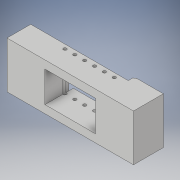
# Autodesk Inventor part: AndersonA
Saved by Autodesk Inventor 2018 (Build 220112000, 112)
## iProperties
Created: 2017-09-11
Part Number: AndersonA
Material: Generic
Document SubType Name: Modeling
Designer: Srinity
Density: 1 g/cm^3
Appearance: Default
Author: Srinity
Autodesk Inventor part; units mm, degrees
ref_plane "YZ Plane" through (0, 0, 0) normal (1, 0, 0) x (0, 1, 0)
ref_plane "XZ Plane" through (0, 0, 0) normal (0, 1, 0) x (-1, 0, 0)
ref_plane "XY Plane" through (0, 0, 0) normal (0, 0, 1) x (1, 0, 0)
derived "Andersonhousing1.ipt"
sketch "Sketch1" plane through (0, 0, 0) normal (0, 0, 1) x (1, 0, 0)
  line L0 (-20.2946, 12.3698) -> (20.2946, 12.3698)
  line L1 (20.2946, 12.3698) -> (20.2946, -12.3698)
  line L2 (20.2946, -12.3698) -> (-20.2946, -12.3698)
  line L3 (-20.2946, -12.3698) -> (-20.2946, 12.3698)
  line L4 (-50.8, 18.7198) -> (50.8, 18.7198)
  line L5 (50.8, 18.7198) -> (50.8, -18.7198)
  line L6 (50.8, -18.7198) -> (-50.8, -18.7198)
  line L7 (-50.8, -18.7198) -> (-50.8, 18.7198)
  circle A0 centre (-17.1196, 15.5448) radius 3.175
  circle A1 centre (17.1196, -15.5448) radius 3.175
  line L8 (20.2946, 12.3698) -> (26.6446, 18.7198)
  line L9 (-20.2946, -12.3698) -> (-26.6446, -18.7198)
  line L10 (19.3966, 12.3698) -> (25.7466, 18.7198)
  line L11 (20.2946, 11.4718) -> (27.5426, 18.7198)
  line L12 (-19.3966, -12.3698) -> (-25.7466, -18.7198)
  line L13 (-20.2946, -11.4718) -> (-27.5426, -18.7198)
  arc A2 (-20.2946, 8.6178) -> (-10.1926, 12.3698) centre (-17.1196, 15.5448) ccw
  arc A3 (10.1926, -12.3698) -> (10.1926, -18.7198) centre (17.1196, -15.5448) ccw
  arc A4 (-14.0087, 12.3698) -> (-20.2305, 12.3698) centre (-17.1196, 15.5448) ccw
  arc A5 (14.0087, -12.3698) -> (20.2305, -12.3698) centre (17.1196, -15.5448) ccw
  arc A6 (-24.0466, 18.7198) -> (-20.2946, 8.6178) centre (-17.1196, 15.5448) ccw
  arc A7 (-10.1926, 18.7198) -> (-24.0466, 18.7198) centre (-17.1196, 15.5448) ccw
  arc A8 (-10.1926, 12.3698) -> (-10.1926, 18.7198) centre (-17.1196, 15.5448) ccw
  arc A9 (20.2946, -8.6178) -> (10.1926, -12.3698) centre (17.1196, -15.5448) ccw
  arc A10 (10.1926, -18.7198) -> (24.0466, -18.7198) centre (17.1196, -15.5448) ccw
  arc A11 (24.0466, -18.7198) -> (20.2946, -8.6178) centre (17.1196, -15.5448) ccw
  arc A12 (20.2305, -12.3698) -> (14.0087, -12.3698) centre (17.1196, -15.5448) ccw
  arc A13 (-20.2305, 12.3698) -> (-14.0087, 12.3698) centre (-17.1196, 15.5448) ccw
  circle A14 centre (-35.5473, -6.0198) radius 6.35
  circle A15 centre (35.5473, 6.0198) radius 6.985
  circle A16 centre (35.5473, 6.0198) radius 6.35 construction
  point P0 (0, 0)
extrude "Extrusion1" add sketch "Sketch1" along normal blind 19.05 contours L3 A6 L4 A4 L0 | A4 L4 A0 L0 | L3 L13 L6 L7 L4 A6 | A0 L4 A4 L0 | A0 | A4 L4 A8 L0 | L3 L9 L6 L13 | A8 L4 L10 L0 | L2 L12 L6 L9 | L10 L4 L8 L0 | L2 A3 L6 L12 | L8 L4 L11 L1 | L2 A5 L6 A3 | L11 L4 L5 L6 A11 L1 | L2 A1 L6 A5 | A11 L6 A5 L2 L1 | L2 A5 L6 A1 | A1 | A14 | A15
extrude "Extrusion2" add sketch "Sketch1" against normal blind 4.953 contours L2 L12 L6 L9 | L2 A3 L6 L12 | L2 A5 L6 A3 | L11 L4 L5 L6 A11 L1 | L2 A1 L6 A5 | A11 L6 A5 L2 L1 | L2 A5 L6 A1 | A1 | A15
chamfer "Chamfer1" distance 1.27 angle 45 4 edges at (0, -12.3698, -4.953) (20.2946, -0.449, -4.953) (-23.4696, -15.5448, -4.953) (23.9186, 15.0958, -4.953)
sketch "Sketch2" plane through (-50.8, 18.7198, 19.05) normal (0, 1, 0) x (1, 0, 0)
  line L0 (30.5054, 19.05) -> (30.5054, 0) projected
  line L1 (30.5054, 19.05) -> (30.5054, 0) projected
  line L2 (71.0946, 0) -> (71.0946, 22.733) projected
  line L3 (71.0946, 19.05) -> (71.0946, 0) projected
  line L4 (71.0946, 19.05) -> (71.0946, 22.733) projected
  circle A0 centre (30.988, 15.5829) radius 1.27
  line L5 (30.5054, 23.3045) -> (45.2822, 23.3045) construction
  circle A1 centre (38.9128, 15.5829) radius 1.27
  circle A2 centre (46.8376, 15.5829) radius 1.27
  circle A3 centre (54.7624, 15.5829) radius 1.27
  circle A4 centre (62.6872, 15.5829) radius 1.27
  circle A5 centre (70.612, 15.5829) radius 1.27
  line L6 (72.3646, 24.003) -> (31.0315, 24.003) projected
  point P0 (50.8, 19.05)
  dimension "d8" = 0.4826
  dimension "d9" = 2.54
  dimension "d12" = 7.9248
  dimension "d17" = 8.4201
  constraints: 6 centre point, 2 end point, 2 horizontal, 1 point on line, 10 other
  measures "d8" distance from line of A0.centre L0
  measures "d9" diameter of A0
  measures "d12" distance of A0.centre A1.centre
  measures "d17" distance from line of A0.centre L6
extrude "Extrusion3" cut sketch "Sketch2" against normal through all
extrude "Extrusion4" add sketch "Sketch1" against normal blind 12.7 contours A14
extrude "Extrusion5" cut sketch "Sketch1" along normal mid plane 25.4 contours A15
chamfer "Chamfer2" distance 1.27 angle 45 1 edges at (28.5623, 6.0198, -4.953)
fillet "Fillet1" radius 3.175 1 edges at (-41.8973, -6.0198, -12.7)
body "Solid1"
